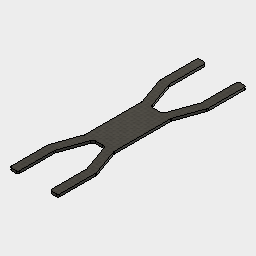
Battery Tray v2 Base (Autodesk Fusion 360 design; units mm, degrees)
Autodesk Fusion 360 part; units mm, degrees
note: some values were not read from the file. Set by a fixed rule: which sketch regions a step uses.
sketch "Sketch1" plane through (0, 0, 0) normal (0, 1, 0) x (1, 0, 0)
  line L0 (14.8, 12) -> (14.8, -8)
  line L1 (-14.8, 12) -> (-14.8, -8)
  line L2 (-9.8, 7) -> (-9.8, -7.0489)
  line L3 (9.8, 7) -> (9.8, -7.0489)
  line L4 (9.8, 7) -> (9.8, 12)
  line L5 (-9.8, 7) -> (-9.8, 12)
  line L6 (14.8, -77.0865) -> (14.8, -97)
  line L7 (-14.8, -77.0873) -> (-14.8, -96.9944)
  line L8 (-9.8, -96.9944) -> (-9.8, -77.9519)
  line L9 (9.8, -97) -> (9.8, -77.9511)
  line L10 (4.0586, -23.6718) -> (9.6258, -8.0563)
  line L11 (-9.0092, -60.3259) -> (-14.6258, -76.0798)
  line L12 (9.0094, -60.3258) -> (14.6258, -76.079)
  line L13 (14.8, -8) -> (14.8, -7.9135)
  line L14 (14.6548, -8.8395) -> (14.6258, -8.921)
  line L15 (-14.6548, -8.8395) -> (-14.6258, -8.921)
  line L16 (-14.8, -7.9135) -> (-14.8, -8)
  line L17 (-4.0585, -23.6718) -> (-9.6258, -8.0563)
  line L18 (-9.6258, -76.9445) -> (-4.0584, -61.3286)
  line L19 (9.0094, -24.6744) -> (14.6548, -8.8395)
  line L20 (9.6258, -76.9437) -> (4.0587, -61.3286)
  line L21 (-9.0092, -24.6747) -> (-14.6548, -8.8395)
  line L22 (-9.8, 12) -> (-9.8, 14)
  line L23 (-14.8, 14) -> (-14.8, 12)
  line L24 (14.8, 12) -> (14.8, 14)
  line L25 (9.8, 14) -> (9.8, 12)
  line L26 (-9.8, -96.9944) -> (-9.8, -98.9944)
  line L27 (-14.8, -98.9944) -> (-14.8, -96.9944)
  line L28 (14.8, -97) -> (14.8, -99)
  line L29 (9.8, -99) -> (9.8, -97)
  line L30 (2.1747, -25.0002) -> (-2.1747, -25.0002)
  line L31 (-8.8931, -25.3464) -> (-8.8931, -59.6542)
  line L32 (-2.1746, -60.0002) -> (2.1748, -60.0002)
  line L33 (8.8933, -59.6541) -> (8.8933, -25.3461)
  arc A0 (-8.8931, -25.3464) -> (-9.0092, -24.6747) centre (-10.8931, -25.3464) ccw
  arc A1 (-4.0585, -23.6718) -> (-2.1747, -25.0002) centre (-2.1747, -23.0002) ccw
  arc A2 (2.1747, -25.0002) -> (4.0586, -23.6718) centre (2.1747, -23.0002) ccw
  arc A3 (9.0094, -24.6744) -> (8.8933, -25.3461) centre (10.8933, -25.3461) ccw
  arc A4 (8.8933, -59.6541) -> (9.0094, -60.3258) centre (10.8933, -59.6541) ccw
  arc A5 (4.0587, -61.3286) -> (2.1748, -60.0002) centre (2.1748, -62.0002) ccw
  arc A6 (-2.1746, -60.0002) -> (-4.0584, -61.3286) centre (-2.1746, -62.0002) ccw
  arc A7 (-9.0092, -60.3259) -> (-8.8931, -59.6542) centre (-10.8931, -59.6542) ccw
  arc A8 (-14.6258, -76.0798) -> (-14.8, -77.0873) centre (-11.8, -77.0873) ccw
  arc A9 (-9.6258, -76.9445) -> (-9.8, -77.9519) centre (-6.8, -77.9519) ccw
  arc A10 (9.8, -77.9511) -> (9.6258, -76.9437) centre (6.8, -77.9511) ccw
  arc A11 (14.8, -77.0865) -> (14.6258, -76.079) centre (11.8, -77.0865) ccw
  arc A12 (14.6258, -8.921) -> (14.8, -7.9135) centre (11.8, -7.9135) ccw
  arc A13 (9.6258, -8.0563) -> (9.8, -7.0489) centre (6.8, -7.0489) ccw
  arc A14 (-9.8, -7.0489) -> (-9.6258, -8.0563) centre (-6.8, -7.0489) ccw
  arc A15 (-14.8, -7.9135) -> (-14.6258, -8.921) centre (-11.8, -7.9135) ccw
  line L34 (-10.8, 15) -> (-13.8, 15)
  line L35 (10.8, 15) -> (13.8, 15)
  line L36 (10.8, -100) -> (13.8, -100)
  line L37 (-10.8, -99.9944) -> (-13.8, -99.9944)
  arc A16 (-14.8, -98.9944) -> (-13.8, -99.9944) centre (-13.8, -98.9944) ccw
  arc A17 (-10.8, -99.9944) -> (-9.8, -98.9944) centre (-10.8, -98.9944) ccw
  arc A18 (9.8, -99) -> (10.8, -100) centre (10.8, -99) ccw
  arc A19 (13.8, -100) -> (14.8, -99) centre (13.8, -99) ccw
  arc A20 (14.8, 14) -> (13.8, 15) centre (13.8, 14) ccw
  arc A21 (-13.8, 15) -> (-14.8, 14) centre (-13.8, 14) ccw
  arc A22 (10.8, 15) -> (9.8, 14) centre (10.8, 14) ccw
  arc A23 (-9.8, 14) -> (-10.8, 15) centre (-10.8, 14) ccw
  point P0 (0.0001, -42.5002)
  dimension "d39" = 1
  measures "d39" radius of A16
extrude "Extrude1" add sketch "Sketch1" along normal blind 1.5
